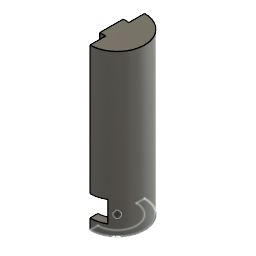
Connector (Autodesk Fusion 360 design; units mm, degrees)
part number: 2026-05-27-14-04-04-217
Autodesk Fusion 360 part; units mm, degrees
sketch "Sketch1" plane through (0, 0, 0) normal (0, 1, 0) x (1, 0, 0)
  arc A0 (0, -23.375) -> (0, 23.375) centre (0, 0) ccw
  arc A1 (0, -23.375) -> (0, 23.375) centre (0, 0) ccw
  arc A2 (0, -16.5) -> (0, 16.5) centre (0, 0) ccw
  line L0 (0, 16.5) -> (0, 23.375)
  line L1 (0, -16.5) -> (0, -23.375)
  constraint coincident A0.centre A1.centre
  constraint coincident A0.end A1.end
  constraint coincident A0.start A1.start
  constraint vertical L0
  constraint parallel L0 L1
  constraint vertical A2.end A0.centre
  constraint vertical A2.start A0.centre
extrude "Extrude1" add sketch "Sketch1" along normal blind 137
sketch "Sketch5" plane through (0, 0, 0) normal (0, -1, 0) x (1, 0, 0)
  arc A0 (0, -16.5) -> (0, 16.5) centre (0, 0) ccw
  line L0 (0, -16.5) -> (0, -23.375)
  arc A1 (0, -23.375) -> (0, 23.375) centre (0, 0) ccw
  line L1 (0, 23.375) -> (0, 16.5)
  line L2 (0, 23.375) -> (0, 16.5)
  line L3 (0, -16.5) -> (0, -23.375)
  arc A2 (0, -16.5) -> (12, -11.324752) centre (0, 0) ccw
  arc A3 (12, 11.324752) -> (0, 16.5) centre (0.050615, 0.117362) ccw
  arc A4 (12, 20.059677) -> (0, 23.375) centre (0, 0) ccw
  arc A5 (0, -23.375) -> (12, -20.059677) centre (0, 0) ccw
  line L4 (12, -11.324752) -> (12, -20.059677)
  line L5 (12, 20.059677) -> (12, 11.324752)
  dimension "d11" = 12
  constraint coincident A1.end L1.start
  constraint coincident A0.end L1.end
  constraint coincident A0.start L0.start
  constraint coincident L0.end A1.start
  constraint concentric A0 A2
  constraint concentric A1 A5
  constraint vertical L5
  constraint vertical L4
extrude "Extrude2" cut sketch "Sketch5" against normal blind 18 from surface at -9 contours A0 L0 A1 L3 A2 A5 L4 | A1 L1 L2 A3 A4 L5 picked at (9.243328, -18.900304) picked at (9.244717, 18.903526)
sketch "Sketch6" plane through (0, 137, 0) normal (0, 1, 0) x (-1, 0, 0)
  arc A0 (0, 16.5) -> (0, -16.5) centre (0, 0) ccw
  line L0 (0, 16.5) -> (0, 23.375)
  arc A1 (0, 23.375) -> (0, -23.375) centre (0, 0) ccw
  line L1 (0, -23.375) -> (0, -16.5)
  arc A2 (0, 16.5) -> (0, -16.5) centre (0, 0) ccw
  line L2 (0, 16.5) -> (0, -16.5)
  constraint coincident A0.end L1.end
  constraint coincident A0.start L0.start
  constraint coincident A0.centre A1.centre
extrude "Extrude3" add sketch "Sketch6" against normal up to surface (54 mm away) contours A0 A2 L2 picked at (-5.582872, -2.68857)
sketch "Sketch7" plane through (0, 0, 0) normal (-1, 0, 0) x (0, 0, 1)
  line L0 (-23.375, 27) -> (-16.5, 27)
  line L1 (-16.5, 27) -> (-16.5, 83)
  line L2 (-16.5, 83) -> (16.5, 83)
  line L3 (16.5, 83) -> (16.5, 27)
  line L4 (16.5, 27) -> (23.375, 27)
  line L5 (23.375, 27) -> (23.375, 137)
  line L6 (23.375, 137) -> (-23.375, 137)
  line L7 (-23.375, 137) -> (-23.375, 27)
  line L8 (-10, 137) -> (10, 137)
  line L9 (10, 137) -> (10, 112)
  line L10 (10, 112) -> (-10, 112)
  line L11 (-10, 112) -> (-10, 137)
  dimension "d18" = 25
  dimension "d19" = 20
  dimension "d20" = 13.375
  constraint horizontal L8
  constraint vertical L9
  constraint horizontal L10
  constraint vertical L11
  constraint coincident L6 L8.start
  measures "d18" distance of L8.end L9.end
  measures "d19" distance of L9.end L10.end
  measures "d20" distance of L5 L9
extrude "Extrude4" add sketch "Sketch7" along normal blind 5 contours L6 L8 L9 L10 L11 picked at (-3.333333, 128.666667)
